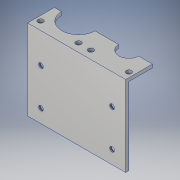
# Autodesk Inventor part: CAR_044_180VersaLBracketMount
Saved by Autodesk Inventor 2018 (Build 220112000, 112)
## iProperties
Created: 2020-02-15
Part Number: CAR_044_180VersaLBracketMount
Material: Aluminum 6061
Document SubType Name: Modeling
Designer: user
Mass: 85.7248 g
Surface Area: 212.701 cm^2
Volume: 31.7499 cm^3
Density: 2.7 g/cm^3
Appearance: Aluminum - Flat
Author: user
Autodesk Inventor part; units mm, degrees
ref_plane "YZ Plane" through (0, 0, 0) normal (1, 0, 0) x (0, 1, 0)
ref_plane "XZ Plane" through (0, 0, 0) normal (0, 1, 0) x (-1, 0, 0)
ref_plane "XY Plane" through (0, 0, 0) normal (0, 0, 1) x (1, 0, 0)
sketch "Sketch1" plane through (0, 0, 0) normal (1, 0, 0) x (0, 1, 0)
  line L0 (0, 0) -> (76.2, 0)
  line L1 (76.2, 0) -> (76.2, -3.175)
  line L2 (76.2, -3.175) -> (0, -3.175)
  line L3 (0, -3.175) -> (0, 0)
  line L4 (76.2, 0) -> (73.025, 0)
  line L5 (73.025, 0) -> (73.025, -25.4)
  line L6 (73.025, -25.4) -> (76.2, -25.4)
  line L7 (76.2, -25.4) -> (76.2, 0)
  dimension "d0" = 76.2
  dimension "d1" = 3.175
  dimension "d2" = 3.175
  dimension "d3" = 25.4
  constraints: 16 end point, 4 parallel, 2 horizontal, 2 perpendicular
  measures "d0" distance of L1.end L2.end
  measures "d1" distance of L2.end L0.start
  measures "d2" distance of L6.end L5.end
  measures "d3" distance of L5.end L4.end
extrude "Extrusion1" add sketch "Sketch1" along normal blind 92.6846
sketch "Sketch2" plane through (0, 76.2, 0) normal (0, 1, 0) x (1, 0, 0)
  line L0 (0, 0) -> (92.6846, 0) projected
  line L1 (0, 25.4) -> (0, 0) projected
  line L2 (46.3423, -68.8852) -> (46.3423, 85.7759) construction
  point P0 (4.5466, 7.7216)
  point P1 (40.4622, 7.7216)
  point P2 (88.138, 7.7216)
  point P3 (52.2224, 7.7216)
  dimension "d6" = 7.7216
  dimension "d7" = 4.5466
  dimension "d8" = 0
  dimension "d9" = 35.9156
  dimension "d27" = 92.6846
  dimension "d28" = 46.3423
  constraints: 2 end point, 2 symmetric about line, 1 vertical
  measures "d6" distance from line of L0 point (4.547, 7.722)
  measures "d7" distance from line of L1 point (4.547, 7.722)
  measures "d8" vertical distance of point (4.547, 7.722) point (40.462, 7.722)
  measures "d9" distance of point (4.547, 7.722) point (40.462, 7.722)
  measures "d27" distance of L0.start L0.end
  measures "d28" distance between parallel lines of L1 L2
hole "Hole1" at (4.5466, 76.2, -7.7216) at (40.4622, 76.2, -7.7216) at (88.138, 76.2, -7.7216) at (52.2224, 76.2, -7.7216) direction (0, -1, 0) diameter 4.9784 depth 25.4 tip angle 118
sketch "Sketch3" plane through (0, 76.2, 0) normal (0, 1, 0) x (1, 0, 0)
  circle A0 centre (22.5044, 25.6794) radius 14.2875 construction
  circle A1 centre (40.4622, 7.7216) radius 2.4892 construction
  point P0 (0, 0)
  dimension "d17" = 28.575
  dimension "d18" = 17.9578
  dimension "d19" = 17.9578
  constraints: 1 centre point, 1 coincident
  measures "d17" diameter of A0
  measures "d18" horizontal distance of A1.centre A0.centre
  measures "d19" horizontal distance of A1.centre A0.centre
hole "Hole2" at (22.5044, 76.2, -25.6794) direction (0, -1, 0) diameter 31.75 depth 25.4 tip angle 118
sketch "Sketch4" plane through (0, 76.2, 0) normal (0, 1, 0) x (1, 0, 0)
  circle A0 centre (88.138, 7.7216) radius 2.4892 projected
  point P0 (0, 0)
  point P1 (70.1802, 25.6794)
  dimension "d29" = 17.9578
  dimension "d30" = 17.9578
  measures "d29" horizontal distance of A0.centre point (70.18, 25.679)
  measures "d30" horizontal distance of A0.centre point (70.18, 25.679)
hole "Hole3" at (70.1802, 76.2, -25.6794) direction (0, -1, 0) diameter 19.05 depth 25.4 tip angle 118
sketch "Sketch5" plane through (0, 0, -3.175) normal (0, 0, -1) x (-1, 0, 0)
  line L0 (0, 0) -> (-92.6846, 0) projected
  line L1 (-92.6846, 0) -> (-92.6846, 73.025) projected
  line L2 (0, 0) -> (0, 73.025) projected
  line L3 (0, 73.025) -> (-6.6319, 73.025) projected
  line L4 (-79.7011, 73.025) -> (-92.6846, 73.025) projected
  point P0 (-79.9846, 47.625)
  point P1 (-12.7, 47.625)
  point P2 (-12.7, 12.7)
  point P3 (-79.9846, 12.7)
  dimension "d38" = 12.7
  dimension "d39" = 12.7
  dimension "d40" = 12.7
  dimension "d41" = 12.7
  dimension "d42" = 12.7
  dimension "d43" = 25.4
  dimension "d44" = 25.4
  dimension "d45" = 12.7
  measures "d38" distance from line of L0 point (-79.985, 12.7)
  measures "d39" distance from line of L1 point (-79.985, 12.7)
  measures "d40" distance from line of L0 point (-12.7, 12.7)
  measures "d41" distance from line of L2 point (-12.7, 12.7)
  measures "d42" distance from line of L2 point (-12.7, 47.625)
  measures "d43" distance from line of L3 point (-12.7, 47.625)
  measures "d44" distance from line of L4 point (-79.985, 47.625)
  measures "d45" distance from line of point (-79.985, 47.625) L1
hole "Hole4" at (79.9846, 47.625, -3.175) at (12.7, 47.625, -3.175) at (12.7, 12.7, -3.175) at (79.9846, 12.7, -3.175) direction (0, 0, 1) diameter 4.4958 end through all countersink diameter 8.4328 countersink angle 82 clearance for "Flat Head Machine Screw (82)" size "#8" standard "Ansi Unified Screw Threads"
equation "\"d28\" = 0.5 * d27"
body "Solid1"
